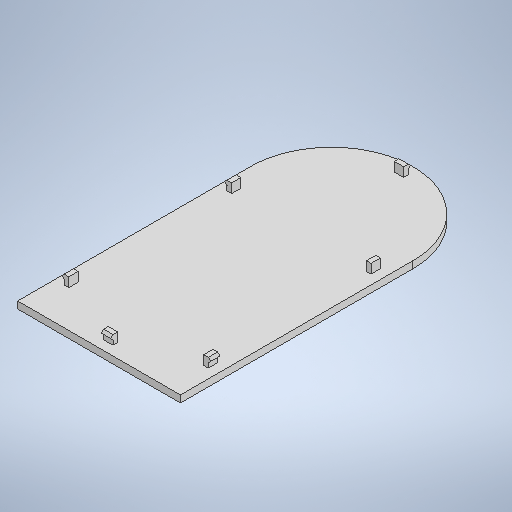
# Autodesk Inventor part: SCARA arm - lid
Saved by Autodesk Inventor 2025.2 (Build 292293000, 293)
## iProperties
Created: 2025-01-29
Part Number: SCARA arm - lid
Material: Generic
Document SubType Name: Modeling
Designer: caomi
Density: 1 g/cm^3
Appearance: Default
Author: caomi
Autodesk Inventor part; units mm, degrees
ref_plane "YZ Plane" through (0, 0, 0) normal (1, 0, 0) x (0, 1, 0)
ref_plane "XZ Plane" through (0, 0, 0) normal (0, 1, 0) x (-1, 0, 0)
ref_plane "XY Plane" through (0, 0, 0) normal (0, 0, 1) x (1, 0, 0)
sketch "Sketch1" plane through (0, 0, 0) normal (0, 1, 0) x (-1, 0, 0)
  line L0 (0, 0) -> (70, 0)
  line L1 (70, 0) -> (70, -100)
  line L2 (70, -100) -> (0, -100)
  line L3 (0, -100) -> (0, 0)
  circle A0 centre (35, -100) radius 35
  point P0 (0, -100)
  dimension "d0" = 70
  dimension "d1" = 100
  constraints: 8 end point, 2 parallel, 1 horizontal, 1 midpoint, 1 perpendicular, 3 other
  measures "d0" distance of L0.start L0.end
  measures "d1" distance of L2.end L0.start
extrude "Extrusion1" add sketch "Sketch1" along normal blind 3
sketch "Sketch3" plane through (0, 3, 0) normal (0, 1, 0) x (1, 0, 0)
  line L0 (-70, 0) -> (0, 0) projected
  line L1 (0, 0) -> (0, 100) projected
  arc A0 (0, 100) -> (-70, 100) centre (-35, 100) ccw projected
  line L2 (-70, 100) -> (-70, 0) projected
  arc A1 (-4, 100) -> (-66, 100) centre (-35, 100) ccw
  line L3 (-4, 100) -> (-4, 4)
  line L4 (-4, 4) -> (-66, 4)
  line L5 (-66, 4) -> (-66, 100)
  arc A2 (-6, 100) -> (-64, 100) centre (-35, 100) ccw
  line L6 (-6, 100) -> (-6, 6)
  line L7 (-6, 6) -> (-64, 6)
  line L8 (-64, 6) -> (-64, 100)
  line L9 (-66, 16) -> (-64, 16)
  line L10 (-64, 16) -> (-64, 20)
  line L11 (-64, 20) -> (-66, 20)
  line L12 (-66, 20) -> (-66, 16)
  line L13 (-78.2924, 53) -> (11.0462, 53) construction
  line L14 (-35, -1.7458) -> (-35, 82.612) construction
  line L15 (-66, 90) -> (-64, 90)
  line L16 (-64, 86) -> (-66, 86)
  line L17 (-4, 16) -> (-6, 16)
  line L18 (-6, 20) -> (-4, 20)
  line L19 (-4, 90) -> (-6, 90)
  line L20 (-6, 86) -> (-4, 86)
  line L21 (-37, 4) -> (-33, 4)
  line L22 (-33, 4) -> (-33, 6)
  line L23 (-33, 6) -> (-37, 6)
  line L24 (-37, 6) -> (-37, 4)
  line L25 (-37, 128.931) -> (-37, 130.9354)
  line L26 (-33, 128.931) -> (-33, 130.9354)
  point P0 (-35, 6)
  point P1 (-64, 53)
  point P2 (-65, 16)
  dimension "d14" = 4
  dimension "d15" = 2
  dimension "d16" = 4
  dimension "d17" = 10
  dimension "d18" = 4
  constraints: 48 end point, 12 symmetric about line, 8 point on circle, 6 point on line, 4 parallel, 3 horizontal, 3 midpoint, 3 vertical, 2 centre point, 2 collinear, 2 perpendicular, 7 other
  measures "d14" distance between parallel lines of L5 L2
  measures "d15" distance between parallel lines of L8 L5
  measures "d16" distance from line of L10.end L9
  measures "d17" distance from line of L7 point (-65, 16)
  measures "d18" distance between parallel lines of L22 L24
extrude "Extrusion2" add sketch "Sketch3" along normal blind 4 contours L26 A2 L25 A1 | L15 L8 L16 L5 | L11 L8 L9 L5 | L4 L24 L7 L22
sketch "Sketch4" plane through (-66, 3, -16) normal (0, 0, 1) x (1, 0, 0)
  line L0 (0, 0) -> (0, 4) projected
  line L1 (0, 4) -> (-1, 3)
  line L2 (-1, 3) -> (0, 2)
  line L3 (-1.3979, 3) -> (0.0465, 3) construction
  point P0 (66, -3)
  dimension "d21" = 1
  dimension "d22" = 45
  constraints: 6 end point, 1 horizontal, 1 midpoint, 1 point on line, 1 other
  measures "d21" distance from line of L0 L1.end
  measures "d22" angle of L2 L3
extrude "Extrusion3" add sketch "Sketch4" against normal up to surface (4 mm away)
extrude "Extrusion4" add sketch "Sketch4" against normal up to surface (4 mm away) from surface at -70
sketch "Sketch5" plane through (-33, 3, -4) normal (1, 0, 0) x (0, 0, -1)
  line L0 (0, 0) -> (0, 4) projected
  line L1 (0, 4) -> (-1, 3)
  line L2 (-1, 3) -> (0, 2)
  line L3 (-1.5711, 3) -> (0, 3) construction
  point P0 (-4, -3)
  dimension "d27" = 1
  dimension "d28" = 45
  constraints: 6 end point, 2 point on line, 1 horizontal, 1 midpoint
  measures "d27" distance from line of L0 L1.end
  measures "d28" angle of L3 L2
extrude "Extrusion5" add sketch "Sketch5" against normal up to surface (4 mm away)
sketch "Sketch6" plane through (-33, 3, -128.931) normal (1, 0, 0) x (0, 0, -1)
  line L0 (2.069, 4) -> (2.0045, 4) projected
  line L1 (2.0045, 4) -> (3.0045, 3)
  line L2 (3.0045, 3) -> (2.0045, 2)
  line L3 (3.5091, 3) -> (1.829, 3) construction
  line L4 (2.0045, 0) -> (2.0045, 4) projected
  point P0 (-128.931, -3)
  dimension "d31" = 45
  dimension "d33" = 1
  constraints: 6 end point, 1 horizontal, 1 midpoint, 1 point on line, 1 other
  measures "d31" angle of L3 L2
  measures "d33" distance from line of L4 L1.end
sketch3d "3D Sketch1"
  arc A0 (-33, 7, -130.9354) -> (-37, 7, -130.9354) centre (-35, 7, -100) ccw
sweep "Sweep1" add profiles "Sketch6" path "3D Sketch1"
ref_plane "Work Plane1" through (-35, 0, -100) normal (-1, 0, 0) x (0, 0, 1)
mirror "Mirror1" about plane through (-35, 0, -100) normal (-1, 0, 0) of "Extrusion2", "Extrusion3"
equation "\"d18\" = d16"
body "Solid1"
